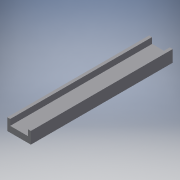
# Autodesk Inventor part: Base
Saved by Autodesk Inventor 2016 (Build 200138000, 138)
## iProperties
Created: 2014-03-12
Part Number: Base
Material: Generic
Document SubType Name: Modeling
Designer: John
Density: 1 g/cm^3
Appearance: Default
Author: John
Autodesk Inventor part; units mm, degrees
ref_plane "YZ Plane" through (0, 0, 0) normal (1, 0, 0) x (0, 1, 0)
ref_plane "XZ Plane" through (0, 0, 0) normal (0, 1, 0) x (-1, 0, 0)
ref_plane "XY Plane" through (0, 0, 0) normal (0, 0, 1) x (1, 0, 0)
sketch "Sketch1" plane through (0, 0, 0) normal (0, 1, 0) x (-1, 0, 0)
  line L0 (12.7, 76.2) -> (-12.7, 76.2)
  line L1 (-12.7, 76.2) -> (-12.7, -76.2)
  line L2 (-12.7, -76.2) -> (12.7, -76.2)
  line L3 (12.7, -76.2) -> (12.7, 76.2)
  line L4 (12.7, 76.2) -> (-12.7, -76.2) construction
  line L5 (-12.7, 76.2) -> (12.7, -76.2) construction
  point P0 (0, 0)
  dimension "d0" = 25.4
  dimension "d1" = 152.4
  constraints: 12 end point, 2 midpoint, 2 parallel, 1 horizontal, 1 perpendicular
  measures "d0" distance of L2.end L1.end
  measures "d1" distance of L1.end L0.end
extrude "Extrusion1" add sketch "Sketch1" along normal blind 12.7
sketch "Sketch2" plane through (-12.7, 0, 76.2) normal (0, 0, 1) x (1, 0, 0)
  line L0 (0, 0) -> (25.4, 0) projected
  line L1 (25.4, 0) -> (25.4, 12.7) projected
  line L2 (0, 12.7) -> (25.4, 12.7) projected
  line L3 (0, 0) -> (0, 12.7) projected
  line L4 (3.175, 12.7) -> (22.225, 12.7)
  line L5 (22.225, 12.7) -> (22.225, 6.35)
  line L6 (22.225, 6.35) -> (3.175, 6.35)
  line L7 (3.175, 6.35) -> (3.175, 12.7)
  point P0 (12.7, 0)
  dimension "d4" = 3.175
  dimension "d5" = 6.35
  dimension "d6" = 3.175
  constraints: 8 end point, 2 parallel, 1 horizontal, 1 perpendicular, 1 point on line
  measures "d4" distance between parallel lines of L1 L5
  measures "d5" distance between parallel lines of L0 L6
  measures "d6" distance between parallel lines of L3 L7
extrude "Extrusion2" cut sketch "Sketch2" against normal through all contours L2 L5 L6 L7
equation "\"d6\" = d4"
body "Solid1"
